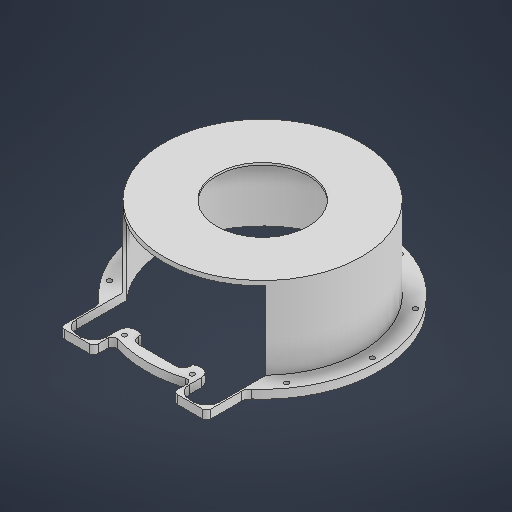
# Autodesk Inventor part: Cylinder  Segment - 01
Saved by Autodesk Inventor 2025 (Build 290162000, 162)
## iProperties
Created: 2024-04-11
Part Number: Cylinder  Segment - 01
Material: Generic
Document SubType Name: Modeling
Designer: Thienan Hoang
Density: 1 g/cm^3
Appearance: Default
Author: Thienan Hoang
Autodesk Inventor part; units mm, degrees
ref_plane "YZ Plane" through (0, 0, 0) normal (1, 0, 0) x (0, 1, 0)
ref_plane "XZ Plane" through (0, 0, 0) normal (0, 1, 0) x (-1, 0, 0)
ref_plane "XY Plane" through (0, 0, 0) normal (0, 0, 1) x (1, 0, 0)
sketch "Sketch1" plane through (0, 0, 0) normal (0, 1, 0) x (-1, 0, 0)
  circle A0 centre (0, 0) radius 135
  circle A1 centre (0, 0) radius 115
  circle A2 centre (0, 0) radius 112.0375
  circle A3 centre (0, 0) radius 9.5
  dimension "Absolute_Diameter" = 270
  dimension "Diameter_No_Outer_Lip" = 230
  dimension "Inner_Cylinder_Diameter" = 224.075
  dimension "Lip_Diameter" = 19
  constraints: 4 centre point, 4 coincident
  measures "Absolute_Diameter" diameter of A0
  measures "Diameter_No_Outer_Lip" diameter of A1
  measures "Inner_Cylinder_Diameter" diameter of A2
  measures "Lip_Diameter" diameter of A3
extrude "Extrusion1" add sketch "Sketch1" along normal blind 10 contours A0
extrude "Extrusion2" add sketch "Sketch1" along normal blind 75 contours A1
sketch "Sketch2" plane through (0, 75, 0) normal (0, 1, 0) x (1, 0, 0)
  circle A0 centre (0, 0) radius 115
  circle A1 centre (0, 0) radius 53.125
  dimension "Lip_Diameter_Out" = 230
  dimension "Inner_Lip_Diameter" = 106.25
  constraints: 2 centre point, 1 coincident
  measures "Lip_Diameter_Out" diameter of A0
  measures "Inner_Lip_Diameter" diameter of A1
extrude "Extrusion7" add sketch "Sketch2" against normal blind 5
ref_plane "Work Plane2" through (0, 10, 0) normal (0, 1, 0) x (1, 0, 0)
sketch "Sketch3" plane through (0, 10, 0) normal (0, 1, 0) x (1, 0, 0)
  circle A0 centre (0, 0) radius 127.5
  circle A1 centre (-127.5, 0) radius 2.75
  circle A2 centre (-103.1497, -74.9426) radius 2.75
  circle A3 centre (-39.3997, -121.2597) radius 2.75
  circle A4 centre (39.3997, -121.2597) radius 2.75
  circle A5 centre (103.1497, -74.9426) radius 2.75
  circle A6 centre (127.5, 0) radius 2.75
  circle A7 centre (103.1497, 74.9426) radius 2.75
  circle A8 centre (39.3997, 121.2597) radius 2.75
  circle A9 centre (-39.3997, 121.2597) radius 2.75
  circle A10 centre (-103.1497, 74.9426) radius 2.75
  dimension "d27" = 255
  dimension "d28" = 5.5
  dimension "d31" = 360
  constraints: 10 centre point, 1 coincident, 1 horizontal alignment, 23 other
  measures "d28" diameter of A1
extrude "Extrusion8" cut sketch "Sketch3" against normal blind 10 contours A0 A6 | A0 A6 | A7 A0 | A0 A7 | A5 A0 | A0 A5 | A8 A0 | A0 A8 | A4 A0 | A0 A4 | A9 A0 | A0 A9 | A3 A0 | A0 A3 | A10 A0 | A0 A10 | A2 A0 | A0 A2 | A1 A0 | A0 A1
chamfer "Chamfer3" [suppressed]
ref_plane "Work Plane6" through (0, 75, 0) normal (0, 1, 0) x (1, 0, 0)
ref_plane "Work Plane11" through (0, 75, 0) normal (0, -1, 0) x (1, 0, 0)
ref_plane "Work Plane10" through (0, 95, 0) normal (0, 1, 0) x (1, 0, 0)
sketch "Sketch8" plane through (0, 95, 0) normal (0, 1, 0) x (1, 0, 0)
  line L0 (-98.5, 3.175) -> (98.5, 3.175)
  line L1 (98.5, 3.175) -> (98.5, -3.175)
  line L2 (98.5, -3.175) -> (-98.5, -3.175)
  line L3 (-98.5, -3.175) -> (-98.5, 3.175)
  line L4 (-98.5, 3.175) -> (98.5, -3.175) construction
  line L5 (98.5, 3.175) -> (-98.5, -3.175) construction
  circle A0 centre (-98.5, 3.175) radius 2.25
  circle A1 centre (-98.5, -3.175) radius 3.75
  circle A2 centre (98.5, 3.175) radius 3.75
  circle A3 centre (98.5, -3.175) radius 3.75
  point P0 (0, 0)
  dimension "d69" = 197
  dimension "d70" = 6.35
  dimension "d71" = 4.5
  dimension "d72" = 7.5
  dimension "d73" = 7.5
  dimension "d74" = 7.5
  constraints: 12 end point, 4 centre point, 4 coincident, 2 midpoint, 2 parallel, 1 horizontal, 1 perpendicular
  measures "d69" distance of L1.end L2.end
  measures "d70" distance of L2.end L0.start
  measures "d71" diameter of A0
  measures "d72" diameter of A1
  measures "d73" diameter of A2
  measures "d74" diameter of A3
hole "Hole2" at (-98.5, 95, -3.175) at (-98.5, 95, 3.175) at (98.5, 95, -3.175) at (98.5, 95, 3.175) direction (0, -1, 0) diameter 3.242 end through all thread size "M4x0.7" class "6H" standard "ANSI Metric M Profile"
hole "Hole3" at (98.5, 95, 3.175) at (98.5, 95, -3.175) at (-98.5, 95, 3.175) at (-98.5, 95, -3.175) direction (0, -1, 0) diameter 7.75 depth 8 tip angle 118
ref_plane "Work Plane7" through (0, 75, 0) normal (0, 1, 0) x (1, 0, 0)
sketch "Sketch12" plane through (0, 75, 0) normal (0, 1, 0) x (1, 0, 0)
  circle A0 centre (0, 0) radius 40
  circle A1 centre (40, 0) radius 1.25
  circle A2 centre (28.2843, 28.2843) radius 1.25
  circle A3 centre (0, 40) radius 1.25
  circle A4 centre (-28.2843, 28.2843) radius 1.25
  circle A5 centre (-40, 0) radius 1.25
  circle A6 centre (-28.2843, -28.2843) radius 1.25
  circle A7 centre (0, -40) radius 1.25
  circle A8 centre (28.2843, -28.2843) radius 1.25
  dimension "d115" = 80
  dimension "d116" = 2.5
  dimension "d119" = 360
  constraints: 8 centre point, 1 coincident, 1 horizontal alignment, 19 other
  measures "d116" diameter of A1
sketch "Sketch13" plane through (0, 0, 0) normal (0, 0, 1) x (1, 0, 0)
  circle A0 centre (0, 45) radius 20.625
  line L0 (134.5, 0) -> (-134.5, 0) projected
  point P0 (0, 0)
  dimension "d128" = 41.25
  dimension "d129" = 45
  constraints: 1 centre point
  measures "d128" diameter of A0
  measures "d129" distance from line of L0 A0.centre
extrude "Extrusion14" cut sketch "Sketch13" along normal through all
extrude "Extrusion15" cut sketch "Sketch12" against normal blind 3 contours A0 A1 | A0 A1 | A2 A0 | A0 A2 | A8 A0 | A0 A8 | A3 A0 | A0 A3 | A7 A0 | A0 A7 | A4 A0 | A0 A4 | A6 A0 | A0 A6 | A5 A0 | A0 A5
ref_plane "Work Plane1" through (0, 10, 0) normal (0, 1, 0) x (1, 0, 0)
sketch "Sketch14" plane through (0, 10, 0) normal (0, 1, 0) x (1, 0, 0)
  circle A0 centre (0, 0) radius 121.0576
  line L0 (-28, -171.0576) -> (28, -171.0576)
  line L1 (28, -171.0576) -> (28, -71.0576)
  line L2 (28, -71.0576) -> (-28, -71.0576)
  line L3 (-28, -71.0576) -> (-28, -171.0576)
  line L4 (-28, -171.0576) -> (28, -71.0576) construction
  line L5 (28, -171.0576) -> (-28, -71.0576) construction
  point P0 (0, -121.0576)
  dimension "d145" = 242.1153
  dimension "d146" = 56
  dimension "d147" = 100
  constraints: 12 end point, 2 midpoint, 2 parallel, 1 horizontal, 1 perpendicular, 1 vertical alignment, 2 other
  measures "d146" distance of L2.end L1.end
  measures "d147" distance of L1.end L0.end
extrude "Extrusion18" cut sketch "Sketch14" along normal blind 55 contours L3 L2 L1 A0 | A0 L1 L0 L3 picked at (0, -87.7243)
ref_plane "Work Plane5" through (0, 0, 0) normal (0, -1, 0) x (1, 0, 0)
sketch "Sketch15" plane through (0, 0, 0) normal (0, -1, 0) x (1, 0, 0)
  circle A0 centre (0, 0) radius 104.7875
  line L0 (22, 122.501) -> (-22, 122.501)
  line L1 (30, 122.501) -> (74, 122.501) construction
  line L2 (30, 114.501) -> (30, 100.4013)
  line L3 (-30, 114.501) -> (-30, 100.4013)
  circle A1 centre (0, 0) radius 53.625 projected
  arc A2 (30, 114.501) -> (22, 122.501) centre (22, 114.501) ccw
  arc A3 (-22, 122.501) -> (-30, 114.501) centre (-22, 114.501) ccw
  point P0 (-30, 122.501)
  point P1 (0, 122.501)
  dimension "d151" = 180
  dimension "d152" = 122.501
  dimension "d153" = 51.1625
  dimension "d154" = 30
  dimension "d155" = 8
  dimension "d159" = 44
  constraints: 8 end point, 6 point on circle, 4 point on line, 4 tangent, 3 centre point, 2 horizontal, 1 coincident, 1 collinear, 1 equal radius, 1 midpoint, 1 parallel, 1 vertical, 1 vertical alignment
  measures "d151" angle of L0 L1
  measures "d152" distance from line of A0.centre L0
  measures "d153" radial gap between concentric circles of A1 A0
  measures "d154" distance from line of point (0, 0) L2
  measures "d155" radius of A2
  measures "d159" distance of L0.start L0.end
extrude "Extrusion19" cut sketch "Sketch15" against normal up to surface (65 mm away) contours A0 L3 A3 L0 A2 L2
ref_plane "Work Plane4" through (0, 0, 0) normal (0, -1, 0) x (1, 0, 0)
sketch "Sketch16" plane through (0, 0, 0) normal (0, -1, 0) x (1, 0, 0)
  circle A0 centre (0, 0) radius 108
  line L0 (-48.125, 96.685) -> (-48.125, 120.7642)
  line L1 (-30, 108.4652) -> (-30, 114.501) projected
  circle A1 centre (0, 0) radius 130
  line L2 (-83.242, 68.8097) -> (-83.242, 99.8537)
  line L3 (-83.242, 68.8097) -> (-48.125, 68.8097)
  line L4 (-48.125, 68.8097) -> (-48.125, 74.6125)
  line L5 (-48.125, 74.6125) -> (-83.242, 74.6125)
  line L6 (-83.242, 74.6125) -> (-83.242, 68.8097)
  line L7 (-48.125, 96.685) -> (-48.125, 68.8097)
  line L8 (48.125, 96.685) -> (48.125, 120.7642)
  line L9 (30, 114.501) -> (30, 108.4652) projected
  line L10 (83.242, 68.8097) -> (83.242, 99.8537)
  circle A2 centre (0, 0) radius 130
  point P0 (-78.0831, 74.6125)
  dimension "d160" = 18.125
  dimension "d163" = 18.125
  dimension "d164" = 35.117
  dimension "d165" = 35.117
  dimension "d166" = 260
  dimension "d167" = 260
  dimension "d170" = 216
  dimension "d181" = 48.125
  constraints: 18 end point, 8 point on circle, 4 parallel, 3 centre point, 3 coincident, 1 collinear, 1 horizontal, 1 perpendicular, 1 vertical
  measures "d160" distance between parallel lines of L1 L0
  measures "d163" distance between parallel lines of L8 L9
  measures "d164" distance of L4.end L5.end
  measures "d165" distance between parallel lines of L8 L10
  measures "d166" diameter of A2
  measures "d167" diameter of A1
  measures "d170" diameter of A0
  measures "d181" distance from line of point (0, 0) L8
extrude "Extrusion21" cut sketch "Sketch16" against normal blind 75 contours A0 L8 A1 L10 | L2 L5 A0 | L5 L2 A1 L0 A0
ref_plane "Work Plane9" through (0, 75, 0) normal (0, 1, 0) x (1, 0, 0)
sketch "Sketch17" plane through (0, 75, 0) normal (0, 1, 0) x (1, 0, 0)
  circle A0 centre (0, 0) radius 115
  line L0 (-51.125, -51.25) -> (-26.125, -51.25)
  line L1 (-26.125, -51.25) -> (-26.125, -96.25)
  line L2 (-26.125, -96.25) -> (-51.125, -96.25)
  line L3 (-51.125, -96.25) -> (-51.125, -51.25)
  line L4 (-51.125, -51.25) -> (-26.125, -96.25) construction
  line L5 (-26.125, -51.25) -> (-51.125, -96.25) construction
  line L6 (-48.125, -104.4461) -> (-48.125, -120.7642) projected
  point P0 (-38.625, -73.75)
  dimension "d171" = 25
  dimension "d172" = 45
  dimension "d173" = 3
  dimension "d174" = 96.25
  constraints: 12 end point, 2 midpoint, 2 parallel, 1 coincident, 1 horizontal, 1 perpendicular, 2 other
  measures "d171" distance of L1.end L2.end
  measures "d172" distance of L0.end L1.end
  measures "d173" distance between parallel lines of L3 L6
  measures "d174" distance from line of point (0, 0) L2
extrude "Extrusion22" cut sketch "Sketch17" against normal blind 10 contours L0 L1 L2 L3
ref_plane "Work Plane8" through (0, 75, 0) normal (0, 1, 0) x (1, 0, 0)
sketch "Sketch18" plane through (0, 75, 0) normal (0, 1, 0) x (1, 0, 0)
  circle A0 centre (0, 0) radius 115
  circle A1 centre (0, 0) radius 53.3681
  dimension "d182" = 230
  constraints: 2 centre point, 2 coincident
  measures "d182" diameter of A0
extrude "Extrusion23" add sketch "Sketch18" along normal mid plane 1
sketch "Sketch20" plane through (0, 75.5, 0) normal (0, 1, 0) x (1, 0, 0)
  circle A0 centre (0, 0) radius 115
  circle A1 centre (0, 0) radius 53.3681
  constraints: 2 centre point, 1 coincident
extrude "Extrusion25" add sketch "Sketch20" along normal blind 30
sketch "Sketch19" plane through (0, 70, 0) normal (0, -1, 0) x (1, 0, 0)
  circle A0 centre (0, 0) radius 112.0375
  constraints: 1 centre point, 1 coincident
extrude "Extrusion24" cut sketch "Sketch19" against normal blind 33
ref_plane "Work Plane3" through (0, 0, 0) normal (0, -1, 0) x (1, 0, 0)
sketch "Sketch21" plane through (0, 0, 0) normal (0, -1, 0) x (1, 0, 0)
  line L0 (83.242, 76.8068) -> (83.242, 99.8537) projected
  line L1 (83.242, 99.8537) -> (48.125, 99.8537)
  line L2 (48.125, 99.8537) -> (48.125, 154.8537)
  line L3 (48.125, 154.8537) -> (83.242, 154.8537)
  line L4 (83.242, 154.8537) -> (83.242, 99.8537)
  line L5 (48.125, 99.8537) -> (83.242, 99.8537)
  line L6 (83.242, 99.8537) -> (83.242, 36.5125)
  line L7 (83.242, 36.5125) -> (48.125, 36.5125)
  line L8 (48.125, 36.5125) -> (48.125, 99.8537)
  line L9 (-48.125, 103.8038) -> (-48.125, 120.7642) projected
  line L10 (-48.125, 120.7642) -> (-83.242, 120.7642)
  line L11 (-83.242, 120.7642) -> (-83.242, 68.9273)
  line L12 (-83.242, 68.9273) -> (-48.125, 68.9273)
  line L13 (-48.125, 68.9273) -> (-48.125, 120.7642)
  line L14 (-48.125, 120.7642) -> (-83.242, 120.7642)
  line L15 (-83.242, 120.7642) -> (-83.242, 153.1873)
  line L16 (-83.242, 153.1873) -> (-48.125, 153.1873)
  line L17 (-48.125, 153.1873) -> (-48.125, 120.7642)
  point P0 (0, 0)
  dimension "d192" = 55
  constraints: 32 end point, 8 parallel, 4 horizontal, 4 perpendicular, 1 point on line
  measures "d192" distance of L1.end L2.end
extrude "Extrusion26" cut sketch "Sketch21" against normal blind 10
sketch "Sketch22" plane through (0, 0, 0) normal (0, -1, 0) x (1, 0, 0)
  circle A0 centre (0, 0) radius 112.0375
  circle A1 centre (0, 0) radius 115
  line L0 (-83.242, 126.1308) -> (-83.242, 73.025)
  line L1 (-83.242, 73.025) -> (-48.125, 73.025)
  line L2 (-48.125, 73.025) -> (-48.125, 126.1308)
  line L3 (-48.125, 116.2458) -> (-48.125, 148.3489)
  line L4 (-48.125, 148.3489) -> (-83.242, 148.3489)
  line L5 (-83.242, 148.3489) -> (-83.242, 126.1308)
  line L6 (-46.125, 124.7457) -> (-46.125, 71.025)
  line L7 (-46.125, 71.025) -> (-85.242, 71.025)
  line L8 (-85.242, 71.025) -> (-85.242, 126.1308)
  line L9 (-85.242, 126.1308) -> (-85.242, 150.3489)
  line L10 (-85.242, 150.3489) -> (-46.125, 150.3489)
  line L11 (-46.125, 150.3489) -> (-46.125, 116.2458)
  line L12 (0, 115) -> (0, 135)
  line L13 (83.242, 126.1308) -> (83.242, 73.025)
  line L14 (83.242, 73.025) -> (48.125, 73.025)
  line L15 (48.125, 73.025) -> (48.125, 126.1308)
  line L16 (48.125, 116.2458) -> (48.125, 148.3489)
  line L17 (48.125, 148.3489) -> (83.242, 148.3489)
  line L18 (83.242, 148.3489) -> (83.242, 126.1308)
  line L19 (46.125, 124.7457) -> (46.125, 71.025)
  line L20 (46.125, 71.025) -> (85.242, 71.025)
  line L21 (85.242, 71.025) -> (85.242, 126.1308)
  line L22 (85.242, 126.1308) -> (85.242, 150.3489)
  line L23 (85.242, 150.3489) -> (46.125, 150.3489)
  line L24 (46.125, 150.3489) -> (46.125, 116.2458)
  point P0 (83.242, 79.3459)
  point P1 (85.242, 77.1933)
  point P2 (-85.242, 77.1933)
  point P3 (-83.242, 79.3459)
  point P4 (46.125, 105.3446)
  point P5 (48.125, 104.4461)
  point P6 (-46.125, 105.3446)
  point P7 (-48.125, 104.4461)
  point P8 (83.242, 74.9878)
  point P9 (48.125, 101.175)
  point P10 (-48.125, 101.175)
  point P11 (-46.125, 102.1023)
  point P12 (-85.242, 72.7063)
  point P13 (-83.242, 74.9878)
  point P14 (46.125, 102.1023)
  point P15 (85.242, 72.7063)
  dimension "d195" = 2
  dimension "d198" = 24.2181
  dimension "d199" = 55.1058
  constraints: 50 end point, 14 symmetric about line, 4 parallel, 2 coincident, 2 point on line, 1 centre point, 8 other
  measures "d195" distance between parallel lines of L5 L9
  measures "d198" distance of L8.end L9.end
  measures "d199" distance of L7.end L8.end
extrude "Extrusion27" add sketch "Sketch22" against normal up to surface (10 mm away) contours A0 L13 A1 L21 | L8 A1 L0 A0 | A1 L13 L18 L17 L16 L15 L19 L24 L23 L22 L21 | L8 L9 L10 L11 L6 A1 L2 L3 L4 L5 L0 | A0 L19 A1 L15 | L2 A1 L6 A0
fillet "Fillet6" radius 5 4 edges at (46.125, 5, 150.3489) (85.242, 5, 150.3489) (-46.125, 5, 150.3489) (-85.242, 5, 150.3489)
fillet "Fillet7" radius 15 4 edges at (48.125, 5, 148.3489) (83.242, 5, 148.3489) (-48.125, 5, 148.3489) (-83.242, 5, 148.3489)
fillet "Fillet8" radius 10 2 edges at (-85.242, 5, 104.6843) (85.242, 5, 104.6843)
extrude "Extrusion28" cut sketch "Sketch16" against normal blind 100 contours A0 L8 A1 L10 | L5 L2 A1 L0 A0
sketch "Sketch23" plane through (0, 0, 0) normal (0, -1, 0) x (1, 0, 0)
  circle A0 centre (0, 0) radius 107.9617
  circle A1 centre (0, 0) radius 115
  line L0 (-48.125, 104.4461) -> (-48.125, 88.194)
  line L1 (48.125, 101.175) -> (48.125, 104.4461) projected
  line L2 (48.125, 104.4461) -> (48.125, 89.9715)
  line L3 (48.125, 89.9715) -> (-48.125, 88.194)
  point P0 (48.125, 96.6422)
  point P1 (-48.125, 96.6422)
  constraints: 6 end point, 2 centre point, 2 coincident, 2 vertical, 1 point on circle
extrude "Extrusion29" cut sketch "Sketch23" against normal up to surface (100 mm away) contours A0 L0 A1 L1 L2 picked at (-43.7453, 101.0747)
fillet "Fillet12" radius 5 2 edges at (-46.125, 5, 126.8759) (46.125, 5, 126.8759)
fillet "Fillet13" radius 10 2 edges at (48.125, 5, 104.4461) (-48.125, 5, 104.4461)
body "Solid1"
